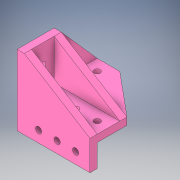
# Autodesk Inventor part: xIdler
Saved by Autodesk Inventor 2019 (Build 230136000, 136)
## iProperties
Created: 2019-05-16
Part Number: xIdler
Material: Generic
Document SubType Name: Modeling
Designer: Alex Jones
Density: 1 g/cm^3
Appearance: Default
Author: Alex Jones
Autodesk Inventor part; units mm, degrees
ref_plane "YZ Plane" through (0, 0, 0) normal (1, 0, 0) x (0, 1, 0)
ref_plane "XZ Plane" through (0, 0, 0) normal (0, 1, 0) x (-1, 0, 0)
sketch "Sketch1" plane through (0, 0, 0) normal (0, 1, 0) x (-1, 0, 0)
  line L0 (-19.05, -19.05) -> (19.05, -19.05) construction
  line L1 (19.05, -19.05) -> (19.05, 19.05) construction
  line L2 (19.05, 19.05) -> (-19.05, 19.05) construction
  line L3 (-19.05, 19.05) -> (-19.05, -19.05) construction
  line L4 (-19.05, -19.05) -> (19.05, 19.05) construction
  line L5 (19.05, -19.05) -> (-19.05, 19.05) construction
  line L6 (-19.05, 19.05) -> (19.05, 19.05) construction
  line L7 (19.05, 19.05) -> (19.05, 39.05) construction
  line L8 (19.05, 39.05) -> (-19.05, 39.05)
  line L9 (-19.05, 39.05) -> (-19.05, 19.05) construction
  line L10 (19.05, 39.05) -> (39.05, 39.05)
  line L11 (39.05, 39.05) -> (39.05, -19.05)
  line L12 (39.05, -19.05) -> (19.05, -19.05) construction
  line L13 (19.05, -19.05) -> (19.05, 19.05) construction
  line L14 (19.05, 19.05) -> (19.05, 39.05) construction
  line L15 (-19.05, 39.05) -> (39.05, 39.05)
  line L16 (45.4, 39.05) -> (45.4, 45.4)
  line L17 (45.4, 45.4) -> (-19.05, 45.4)
  line L18 (-19.05, 45.4) -> (-19.05, 39.05)
  line L19 (45.4, 39.05) -> (39.05, 39.05) construction
  line L20 (39.05, 39.05) -> (39.05, -19.05)
  line L21 (39.05, -19.05) -> (45.4, -19.05)
  line L22 (45.4, -19.05) -> (45.4, 39.05)
  line L23 (39.05, 39.05) -> (45.4, 39.05) construction
  point P0 (0, 0)
  dimension "d0" = 38.1
  dimension "d1" = 20
  dimension "d2" = 20
  dimension "d3" = 6.35
  dimension "d4" = 6.35
  dimension "d67" = 0
  constraints: 48 end point, 12 parallel, 7 perpendicular, 6 horizontal, 2 midpoint
  measures "d0" distance of L0.end L1.end
  measures "d1" distance of L11.end L12.end
  measures "d2" distance of L8.end L2.end
  measures "d3" distance of L11.end L21.end
  measures "d4" distance of L17.end L8.end
  measures "d67" distance between parallel lines of L0 L21
extrude "Extrusion1" add sketch "Sketch1" along normal blind 62.3
sketch "Sketch2" plane through (-45.4, 0, 45.4) normal (0, 0, 1) x (1, 0, 0)
  line L0 (6.35, 0) -> (0, 0) projected
  line L1 (64.45, 0) -> (64.45, 62.3) projected
  line L2 (0, 0) -> (64.45, 0)
  line L3 (64.45, 0) -> (64.45, 20)
  line L4 (64.45, 20) -> (0, 20)
  line L5 (0, 20) -> (0, 0)
  line L6 (0, 0) -> (0, 62.3) projected
  line L7 (0, 10) -> (64.45, 10) construction
  circle A0 centre (19.05, 10) radius 2.75
  circle A1 centre (35.4, 10) radius 2.75
  circle A2 centre (51.75, 10) radius 2.75
  point P0 (45.4, 0)
  dimension "d7" = 20
  dimension "d8" = 5.5
  dimension "d12" = 16.35
  dimension "d68" = 12.7
  constraints: 10 end point, 3 centre point, 3 point on line, 2 horizontal, 2 parallel, 1 midpoint, 1 perpendicular, 4 other
  measures "d7" distance between parallel lines of L2 L4
  measures "d8" diameter of A0
  measures "d12" distance of A0.centre A1.centre
  measures "d68" distance from line of L1 A2.centre
extrude "Extrusion2" cut sketch "Sketch2" against normal blind 62.3 contours A0 | A1 | A2
sketch "Sketch3" plane through (-45.4, 0, -19.05) normal (-1, 0, 0) x (0, 0, 1)
  circle A0 centre (12.7, 10) radius 2.75
  line L0 (0, 0) -> (64.45, 0) projected
  line L1 (0, 0) -> (0, 62.3) projected
  circle A1 centre (29.05, 10) radius 2.75
  circle A2 centre (45.4, 10) radius 2.75
  point P0 (19.05, 0)
  dimension "d19" = 10
  dimension "d20" = 5.5
  dimension "d21" = 12.7
  dimension "d24" = 16.35
  constraints: 3 centre point, 1 horizontal, 4 other
  measures "d19" distance from line of L0 A0.centre
  measures "d20" diameter of A0
  measures "d21" distance from line of L1 A0.centre
  measures "d24" distance of A0.centre A1.centre
extrude "Extrusion3" cut sketch "Sketch3" against normal blind 62.3
ref_plane "Work Plane1" through (0, 20, 0) normal (0, -1, 0) x (1, 0, 0)
sketch "Sketch4" plane through (0, 20, 0) normal (0, -1, 0) x (1, 0, 0)
  line L0 (-39.05, -19.05) -> (-45.4, -19.05) projected
  line L1 (-39.05, 39.05) -> (-39.05, -19.05) projected
  line L2 (19.05, 39.05) -> (-39.05, 39.05) projected
  line L3 (19.05, 45.4) -> (19.05, 39.05) projected
  line L4 (-45.4, 45.4) -> (19.05, 45.4) projected
  line L5 (-45.4, -19.05) -> (-45.4, 45.4) projected
  line L6 (-39.05, 39.05) -> (-39.05, -19.05) projected
  line L7 (-39.05, 39.05) -> (-19.05, 39.05)
  line L8 (-19.05, 39.05) -> (-19.05, 19.05) construction
  line L9 (-19.05, -19.05) -> (-39.05, -19.05)
  line L10 (-39.05, -19.05) -> (-39.05, 39.05)
  line L11 (19.05, 39.05) -> (-39.05, 39.05) projected
  line L12 (19.05, 39.05) -> (-19.05, 39.05)
  line L13 (-19.05, 39.05) -> (-19.05, 19.05) construction
  line L14 (-19.05, 19.05) -> (19.05, 19.05) construction
  line L15 (19.05, 19.05) -> (19.05, 39.05)
  line L16 (-19.05, 19.05) -> (-19.05, -19.05) construction
  line L17 (19.05, 29.05) -> (-39.05, 29.05) construction
  line L18 (-29.05, -19.05) -> (-29.05, 39.05) construction
  circle A0 centre (-29.05, 29.05) radius 2.75
  circle A1 centre (-10, 29.05) radius 2.75
  circle A2 centre (9.05, 29.05) radius 2.75
  circle A3 centre (-29.05, 10) radius 2.75
  circle A4 centre (-29.05, -9.05) radius 2.75
  line L19 (19.05, 19.05) -> (19.05, 12.7)
  line L20 (19.05, 12.7) -> (-19.05, -19.05)
  circle A5 centre (-29.05, 4.126) radius 2.7544
  point P0 (0, 0)
  dimension "d32" = 20
  dimension "d35" = 19.05
  dimension "d40" = 5.5
  dimension "d43" = 19.05
  dimension "d50" = 6.35
  dimension "d69" = 0
  constraints: 26 end point, 6 centre point, 6 perpendicular, 5 parallel, 5 point on line, 3 horizontal, 2 midpoint, 2 vertical, 8 other
  measures "d32" distance of L14.end L2.start
  measures "d35" distance of A0.centre A1.centre
  measures "d40" diameter of A0
  measures "d43" distance of A0.centre A3.centre
  measures "d50" distance of L14.end L19.end
  measures "d69" distance between parallel lines of L0 L9
extrude "Extrusion4" add sketch "Sketch4" against normal blind 6.35 contours L1 L2 L15 L19 L20 L9 | A3
sketch "Sketch5" plane through (0, 26.35, 0) normal (0, 1, 0) x (1, 0, 0)
  line L0 (19.05, -39.05) -> (19.05, -12.7) projected
  line L1 (-39.05, -39.05) -> (-39.05, 19.05) projected
  line L2 (19.05, -12.7) -> (-39.05, -12.7)
  line L3 (-39.05, -12.7) -> (-39.05, -19.05)
  line L4 (-39.05, -19.05) -> (19.05, -19.05)
  line L5 (19.05, -19.05) -> (19.05, -12.7)
  point P0 (0, 0)
  dimension "d51" = 6.35
  constraints: 8 end point, 2 parallel, 1 horizontal, 1 perpendicular, 1 point on line
  measures "d51" distance between parallel lines of L4 L2
extrude "Extrusion5" add sketch "Sketch5" along normal up to surface (35.95 mm away)
sketch "Sketch7" plane through (-39.05, 26.35, -19.05) normal (1, 0, 0) x (0, 0, -1)
  line L0 (-31.75, 35.95) -> (0, 35.95) projected
  line L1 (-31.75, 35.95) -> (0, 35.95)
  line L2 (0, 0) -> (0, 35.95) projected
  line L3 (0, 35.95) -> (0, 0)
  line L4 (0, 0) -> (-31.75, 35.95)
  point P0 (-19.05, -26.35)
  constraints: 6 end point, 1 collinear, 1 perpendicular
extrude "Extrusion7" cut sketch "Sketch7" against normal through all
sketch "Sketch8" plane through (-45.4, 0, 45.4) normal (0, 0, 1) x (1, 0, 0)
  line L0 (64.45, 62.3) -> (6.35, 62.3) projected
  line L1 (6.35, 26.35) -> (6.35, 62.3) projected
  line L2 (64.45, 26.35) -> (6.35, 26.35) projected
  line L3 (64.45, 26.35) -> (64.45, 62.3) projected
  line L4 (64.45, 20) -> (64.45, 26.35) projected
  line L5 (6.35, 62.3) -> (64.45, 26.35)
  line L6 (6.35, 62.3) -> (64.45, 62.3) projected
  line L7 (64.45, 26.35) -> (64.45, 62.3)
  line L8 (64.45, 62.3) -> (6.35, 62.3)
  point P0 (45.4, 0)
  constraints: 6 end point, 2 perpendicular
extrude "Extrusion8" cut sketch "Sketch8" against normal through all contours L3 L5 L0
sketch "Sketch9" plane through (-39.05, 26.35, 39.05) normal (1, 0, 0) x (0, 0, -1)
  line L0 (12.75, -6.35) -> (7.25, -6.35) projected
  line L1 (10, -6.35) -> (10, 18.61)
  circle A0 centre (10, 18.61) radius 2.75
  point P0 (39.05, -26.35)
  dimension "d63" = 24.96
  dimension "d64" = 5.5
  constraints: 2 end point, 1 centre point, 1 coincident, 1 midpoint, 1 vertical
  measures "d63" distance of L1.start L1.end
  measures "d64" diameter of A0
extrude "Extrusion9" cut sketch "Sketch9" against normal through all
body "Solid1"
